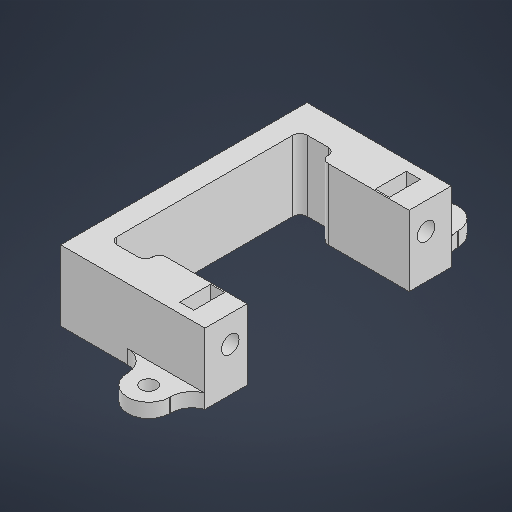
# Autodesk Inventor part: Servo Holder
Saved by Autodesk Inventor 2025.1 (Build 291241000, 241)
## iProperties
Created: 2025-03-13
Part Number: Servo Holder
Material: Generic
Document SubType Name: Modeling
Designer: jerem
Density: 1 g/cm^3
Appearance: Default
Author: jerem
## iProperties of the stored document Servo Holder_3DPrint.ipt
Created: 2025-03-13
Part Number: Servo Holder_3DPrint
Material: Generic
Document SubType Name: Modeling
Designer: jerem
Density: 1 g/cm^3
Appearance: Default
Author: jerem
Autodesk Inventor part; units mm, degrees
ref_plane "YZ Plane" through (0, 0, 0) normal (1, 0, 0) x (0, 1, 0)
ref_plane "XZ Plane" through (0, 0, 0) normal (0, 1, 0) x (-1, 0, 0)
ref_plane "XY Plane" through (0, 0, 0) normal (0, 0, 1) x (1, 0, 0)
sketch "Sketch1" plane through (0, 0, 0) normal (0, 1, 0) x (-1, 0, 0)
  line L0 (0, 17.5) -> (0, 11.5)
  line L1 (0, 11.5) -> (17.5, 11.5)
  line L2 (17.5, 11.5) -> (17.5, 0)
  line L3 (17.5, 0) -> (17.5, -11.5)
  line L4 (17.5, -11.5) -> (0, -11.5)
  line L5 (0, -11.5) -> (0, -17.5)
  line L6 (0, -17.5) -> (20.5, -17.5)
  line L7 (20.5, -17.5) -> (20.5, 17.5)
  line L8 (20.5, 17.5) -> (0, 17.5)
  line L9 (0, 0) -> (0, 11.5) construction
  line L10 (0, 0) -> (0, -11.5) construction
  line L11 (8, 17.5) -> (8, 23.5)
  line L12 (8, 23.5) -> (2, 23.5)
  line L13 (2, 23.5) -> (2, 17.5)
  line L14 (2, -17.5) -> (2, -23.5)
  line L15 (2, -23.5) -> (8, -23.5)
  line L16 (8, -23.5) -> (8, -17.5)
  circle A0 centre (5, 20.5) radius 1.1
  circle A1 centre (5, -20.5) radius 1.1
  line L17 (5, 20.5) -> (5, 23.5) construction
  line L18 (5, -20.5) -> (5, -23.5) construction
  line L19 (5, -20.5) -> (5, 20.5) construction
  line L20 (17.5, 11.5) -> (17.5, 13.5)
  line L21 (17.5, 13.5) -> (12.5, 13.5)
  line L22 (12.5, 13.5) -> (12.5, 11.5)
  line L23 (17.5, -11.5) -> (17.5, -13.5)
  line L24 (17.5, -13.5) -> (12.5, -13.5)
  line L25 (12.5, -13.5) -> (12.5, -11.5)
  dimension "d0" = 23
  dimension "d1" = 17.5
  dimension "d2" = 3
  dimension "d4" = 6
  dimension "d16" = 2.2
  dimension "d17" = 2.2
  dimension "d18" = 3
  dimension "d19" = 3
  dimension "d24" = 41
  dimension "d26" = 5
  dimension "d27" = 5
  dimension "d28" = 2
  constraints: 52 end point, 17 perpendicular, 12 point on line, 7 equal length, 6 vertical, 2 centre point, 2 midpoint
  measures "d0" distance between parallel lines of L4 L1
  measures "d1" distance of L0.end L1.end
  measures "d2" distance between parallel lines of L2 L7
  measures "d4" distance of L0.start L0.end
  measures "d16" diameter of A0
  measures "d17" diameter of A1
  measures "d18" distance between parallel lines of L11 L17
  measures "d19" distance of L17.start L17.end
  measures "d24" distance of L18.start L17.start
  measures "d26" distance between parallel lines of L10 L19
  measures "d27" distance of L20.end L21.end
  measures "d28" distance of L1.end L20.end
extrude "Extrusion1" add sketch "Sketch1" along normal blind 10 contours L8 L7 L6 L5 L4 L25 L24 L23 L3 L2 L20 L21 L22 L1 L0
sketch "Sketch2" plane through (0, 0, 17.5) normal (1, 0, 0) x (0, 0, -1)
  line L0 (6, 0) -> (6, 10) projected
  line L1 (0, 10) -> (6, 10) projected
  line L2 (0, 0) -> (0, 10) projected
  line L3 (35, 0) -> (35, 10) projected
  line L4 (29, 10) -> (35, 10) projected
  line L5 (29, 0) -> (29, 10) projected
  circle A0 centre (3.6, 6.2) radius 1.25
  circle A1 centre (31.4, 6.2) radius 1.25
  line L6 (3.6, 6.2) -> (3.6, 0) construction
  line L7 (31.4, 6.2) -> (31.4, 0) construction
  line L8 (6, 0) -> (3.6, 0) construction
  line L9 (29, 0) -> (31.4, 0) construction
  line L10 (3.6, 6.2) -> (6, 6.2) construction
  line L11 (31.4, 6.2) -> (29, 6.2) construction
  point P0 (17.5, 0)
  dimension "d7" = 2.5
  dimension "d31" = 27.8
  dimension "d33" = 6.2
  constraints: 12 end point, 3 perpendicular, 3 point on line, 2 centre point, 2 equal length, 1 equal radius, 1 vertical
  measures "d7" diameter of A0
  measures "d31" distance between parallel lines of L7 L6
  measures "d33" distance of L6.start L6.end
extrude "Extrusion2" cut sketch "Sketch2" against normal blind 10
sketch "Sketch3" plane through (0, 10, 0) normal (0, 1, 0) x (1, 0, 0)
  line L0 (0, -11.5) -> (-12.5, -11.5) projected
  line L1 (-17.5, -13.5) -> (-17.5, 13.5) projected
  line L2 (-12.5, 11.5) -> (0, 11.5) projected
  line L3 (0, 17.5) -> (-20.5, 17.5) projected
  line L4 (-20.5, 17.5) -> (-20.5, -17.5) projected
  line L5 (-20.5, -17.5) -> (0, -17.5) projected
  line L6 (-3, -11.7) -> (-5, -11.7)
  line L7 (-5, -11.7) -> (-5, -16.1)
  line L8 (-5, -16.1) -> (-3, -16.1)
  line L9 (-3, -16.1) -> (-3, -11.7)
  line L10 (-3, -11.7) -> (-5, -16.1) construction
  line L11 (-5, -11.7) -> (-3, -16.1) construction
  line L12 (-3, 16.1) -> (-5, 16.1)
  line L13 (-5, 16.1) -> (-5, 11.7)
  line L14 (-5, 11.7) -> (-3, 11.7)
  line L15 (-3, 11.7) -> (-3, 16.1)
  line L16 (-3, 16.1) -> (-5, 11.7) construction
  line L17 (-5, 16.1) -> (-3, 11.7) construction
  line L18 (-12.5, -11.5) -> (-12.5, -13.5) projected
  line L19 (-12.5, -13.5) -> (-17.5, -13.5) projected
  line L20 (-17.5, 13.5) -> (-12.5, 13.5) projected
  line L21 (-12.5, 13.5) -> (-12.5, 11.5) projected
  line L22 (0, -12.65) -> (0, -15.15) projected
  line L23 (0, 15.15) -> (0, 12.65) projected
  line L24 (0, 13.9) -> (-3, 13.9) construction
  line L25 (-3, -13.9) -> (0, -13.9) construction
  point P0 (0, 0)
  dimension "d11" = 4.4
  dimension "d13" = 2
  dimension "d34" = 3
  constraints: 28 end point, 4 midpoint, 4 parallel, 4 perpendicular, 2 equal length, 2 horizontal, 1 point on line
  measures "d11" distance of L6.end L7.end
  measures "d13" distance of L6.start L6.end
  measures "d34" distance between parallel lines of L9 L22
extrude "Extrusion3" cut sketch "Sketch3" against normal blind 7
extrude "Extrusion4" add sketch "Sketch1" along normal blind 2 contours L13 L12 L11 L8 | L16 L15 L14 L6
fillet "Fillet1" radius 3 8 edges at (-2, 1, 17.5) (-2, 1, -17.5) (-8, 1, 17.5) (-8, 1, -17.5) (-2, 1, 23.5) (-8, 1, 23.5) (-8, 1, -23.5) (-2, 1, -23.5)
fillet "Fillet2" radius 1 6 edges at (-17.5, 5, 13.5) (-12.5, 5, 13.5) (-12.5, 5, 11.5) (-17.5, 5, -13.5) (-12.5, 5, -13.5) (-12.5, 5, -11.5)
body "Solid1"
